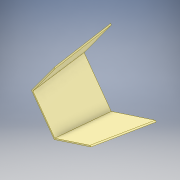
# Autodesk Inventor part: 花盆主体
Saved by Autodesk Inventor 2018 (Build 220112000, 112)
## iProperties
Created: 2021-02-25
Part Number: 花盆主体
Material: 尼龙 6/6
Document SubType Name: Modeling
Designer: OHHHHHHHHHH
Density: 1.13 g/cm^3
Appearance: 尼龙 6
Author: OHHHHHHHHHH
Autodesk Inventor part; units mm, degrees
sketch "草图1" plane through (0, 0, 0) normal (0, 1, 0) x (-1, 0, 0)
  line L0 (82.5131, 0) -> (25.498, -78.4746)
  line L1 (25.498, -78.4746) -> (-66.7545, -48.5)
  line L2 (-66.7545, -48.5) -> (-66.7545, 48.5)
  line L3 (-66.7545, 48.5) -> (25.498, 78.4746)
  line L4 (25.498, 78.4746) -> (82.5131, 0)
  point P0 (0, 0)
  point P1 (0, 0)
  dimension "d0" = 97
  constraints: 10 end point, 1 coincident, 11 other
  measures "d0" distance of L1.end L2.end
ref_plane "工作平面1" through (0, 170, 0) normal (0, 1, 0) x (-1, 0, 0)
sketch "草图2" plane through (0, 170, 0) normal (0, 1, 0) x (-1, 0, 0)
  line L0 (105.0554, 0) -> (32.4639, -99.9136)
  line L1 (32.4639, -99.9136) -> (-84.9916, -61.75)
  line L2 (-84.9916, -61.75) -> (-84.9916, 61.75)
  line L3 (-84.9916, 61.75) -> (32.4639, 99.9136)
  line L4 (32.4639, 99.9136) -> (105.0554, 0)
  point P0 (0, 0)
  point P1 (0, 0)
  dimension "d2" = 123.5
  constraints: 10 end point, 1 coincident, 11 other
  measures "d2" distance of L1.end L2.end
loft "放样1" add profiles "草图2", "草图1"
sketch "草图3" plane through (84.9916, 170, 61.75) normal (0, 1, 0) x (1, 0, 0)
  line L0 (-153.2988, 61.75) -> (-106.0997, 126.7141)
  line L1 (-106.0997, 126.7141) -> (-29.7298, 101.9)
  line L2 (-29.7298, 101.9) -> (-29.7298, 21.6)
  line L3 (-29.7298, 21.6) -> (-106.0997, -3.2141)
  line L4 (-106.0997, -3.2141) -> (-153.2988, 61.75)
  point P0 (-84.9916, 61.75)
  point P1 (-84.9916, 61.75)
  dimension "d7" = 80.3
  constraints: 10 end point, 1 coincident, 11 other
  measures "d7" distance of L1.end L2.end
extrude "拉伸1" cut sketch "草图3" against normal blind 164
shell "抽壳1" thickness 3 removed faces 1 at (10.4732, 170, -75.5426)
sketch "草图5" plane through (66.7545, 0, -48.5) normal (0, -1, 0) x (1, 0, 0)
  line L0 (-98.0659, 144.8667) -> (-91.2229, 123.806) projected
  line L1 (-106.5917, 71.5) -> (-123.9122, 81.5)
  line L2 (-107.7408, 69.3836) -> (-125.561, 78.4634)
  arc A0 (-106.5917, 71.5) -> (-107.7408, 69.3836) centre (-66.7545, 48.5) ccw
  arc A1 (-123.9122, 81.5) -> (-125.561, 78.4634) centre (-66.7545, 48.5) ccw
  point P0 (-99.2814, 81.0269)
  dimension "d37" = 132
  dimension "d38" = 92
  dimension "d40" = 3
  constraints: 5 point on circle, 4 end point, 2 centre point, 1 coincident
  measures "d37" diameter of A1
  measures "d38" diameter of A0
  measures "d40" angle of L1 L2
extrude "拉伸2" add sketch "草图5" along normal blind 3
sketch "草图7" plane through (66.7545, -3, -48.5) normal (0, -1, 0) x (1, 0, 0)
  arc A0 (-100.9392, 79.28) -> (-106.5917, 71.5) centre (-66.7545, 48.5) ccw
  arc A1 (-115.8021, 92.6626) -> (-125.561, 78.4634) centre (-66.7545, 48.5) ccw
  arc A2 (-100.9392, 79.28) -> (-107.7408, 69.3836) centre (-66.7545, 48.5) ccw
  line L0 (-100.9392, 79.28) -> (-115.8021, 92.6626)
  line L1 (-125.561, 78.4634) -> (-107.7408, 69.3836) projected
  line L2 (-107.7408, 69.3836) -> (-125.561, 78.4634)
  dimension "d25" = 92
  dimension "d41" = 15
  constraints: 6 point on circle, 4 end point, 3 centre point, 1 coincident, 1 collinear
  measures "d25" diameter of A0
  measures "d41" angle of L2 L0
extrude "拉伸3" add sketch "草图7" along normal blind 3
chamfer "倒角1" distance 1 angle 45 1 edges at (-41.6161, -3, 37.4713)
sketch "草图8" plane through (66.7545, 0, -48.5) normal (0, -1, 0) x (1, 0, 0)
  circle A0 centre (-66.7545, 48.5) radius 15
  dimension "d100" = 30
  constraints: 1 centre point, 1 coincident
  measures "d100" diameter of A0
extrude "拉伸4" add sketch "草图8" along normal blind 30
pattern_circular "环形阵列1" count 10 over 360 about axis through (0, -10, 0) along (0, 1, 0) of "拉伸3", "拉伸2", "倒角1"
sketch "草图9" plane through (64.0591, 3, 46.5417) normal (0, 1, 0) x (1, 0, 0)
  line L0 (-132.3664, 46.5417) -> (-85.1672, 111.5058) projected
  line L1 (-85.1672, -18.4224) -> (-132.3664, 46.5417) projected
  line L2 (-8.7974, 6.3917) -> (-85.1672, -18.4224) projected
  line L3 (-8.7974, 86.6917) -> (-8.7974, 6.3917) projected
  line L4 (-85.1672, 111.5058) -> (-8.7974, 86.6917) projected
  line L5 (-136.0746, 46.5417) -> (-86.3131, -21.9491) projected
  line L6 (-86.3131, -21.9491) -> (-5.7974, 4.2121) projected
  line L7 (-5.7974, 4.2121) -> (-5.7974, 88.8713) projected
  line L8 (-5.7974, 88.8713) -> (-86.3131, 115.0325) projected
  line L9 (-86.3131, 115.0325) -> (-136.0746, 46.5417) projected
  line L10 (-85.1672, -18.4224) -> (-132.3664, 46.5417) projected
  line L11 (-132.3664, 46.5417) -> (-85.1672, 111.5058) projected
  line L12 (-85.1672, 111.5058) -> (-8.7974, 86.6917) projected
  line L13 (-8.7974, 86.6917) -> (-8.7974, 6.3917) projected
  line L14 (-8.7974, 6.3917) -> (-85.1672, -18.4224) projected
  line L15 (-143.2406, 46.5417) -> (-88.5276, 121.8477) projected
  line L16 (-88.5276, -28.7643) -> (-143.2406, 46.5417) projected
  line L17 (0, 0) -> (-88.5276, -28.7643) projected
  line L18 (0, 93.0834) -> (0, 0) projected
  line L19 (-88.5276, 121.8477) -> (0, 93.0834) projected
  line L20 (-145.4076, 46.5417) -> (-89.1972, 123.9087)
  line L21 (-89.1972, 123.9087) -> (1.7532, 94.3571)
  line L22 (1.7532, 94.3571) -> (1.7532, -1.2738)
  line L23 (1.7532, -1.2738) -> (-89.1972, -30.8253)
  line L24 (-89.1972, -30.8253) -> (-145.4076, 46.5417)
  point P0 (-64.0591, 46.5417)
  constraints: 10 end point, 4 other
extrude "拉伸5" add sketch "草图9" along normal blind 15 contours L15 L19 L18 L17 L16 | L20 L21 L22 L23 L24
sketch "草图10" plane through (84.9916, 6, 61.75) normal (0, 1, 0) x (1, 0, 0)
  line L0 (-153.2988, 61.75) -> (-106.0997, 126.7141) projected
  line L1 (-106.0997, -3.2141) -> (-153.2988, 61.75) projected
  line L2 (-29.7298, 21.6) -> (-106.0997, -3.2141) projected
  line L3 (-29.7298, 101.9) -> (-29.7298, 21.6) projected
  line L4 (-106.0997, 126.7141) -> (-29.7298, 101.9) projected
  line L5 (-107.2456, 130.2408) -> (-157.007, 61.75) projected
  line L6 (-26.7298, 104.0796) -> (-107.2456, 130.2408) projected
  line L7 (-26.7298, 19.4204) -> (-26.7298, 104.0796) projected
  line L8 (-107.2456, -6.7408) -> (-26.7298, 19.4204) projected
  line L9 (-157.007, 61.75) -> (-107.2456, -6.7408) projected
  line L10 (-166.1621, 61.75) -> (-110.0746, 138.9477) projected
  line L11 (-110.0746, -15.4477) -> (-166.1621, 61.75) projected
  line L12 (-19.3233, 14.0392) -> (-110.0746, -15.4477) projected
  line L13 (-19.3233, 109.4608) -> (-19.3233, 14.0392) projected
  line L14 (-110.0746, 138.9477) -> (-19.3233, 109.4608) projected
  point P0 (-84.9916, 61.75)
sketch "草图11" plane through (64.0591, 18, 46.5417) normal (0, 1, 0) x (1, 0, 0)
  line L0 (-64.0591, 46.5417) -> (2.6954, 46.5417) construction
  line L1 (-86.3131, 115.0325) -> (-136.0746, 46.5417) projected
  line L2 (-5.7974, 88.8713) -> (-86.3131, 115.0325) projected
  line L3 (-5.7974, 4.2121) -> (-5.7974, 88.8713) projected
  line L4 (-86.3131, -21.9491) -> (-5.7974, 4.2121) projected
  line L5 (-136.0746, 46.5417) -> (-86.3131, -21.9491) projected
  line L6 (-145.2296, 46.5417) -> (-89.1422, 123.7394) projected
  line L7 (-89.1422, -30.656) -> (-145.2296, 46.5417) projected
  line L8 (1.6092, -1.1691) -> (-89.1422, -30.656) projected
  line L9 (1.6092, 94.2525) -> (1.6092, -1.1691) projected
  line L10 (-89.1422, 123.7394) -> (1.6092, 94.2525) projected
  circle A0 centre (-2.0908, 11.2121) radius 1.25
  line L11 (-5.7974, 4.2121) -> (1.6092, -1.1691) construction
  line L12 (-5.7974, 4.2121) -> (-5.7974, 88.8713) projected
  line L13 (-86.3131, -21.9491) -> (-5.7974, 4.2121) projected
  line L14 (1.6092, -1.1691) -> (-89.1422, -30.656) projected
  line L15 (1.6092, 94.2525) -> (1.6092, -1.1691) projected
  circle A1 centre (-11.3094, -1.4762) radius 1.25
  line L16 (-2.0941, 7.5215) -> (-0.5941, 7.5215)
  line L17 (-0.5941, 7.5215) -> (-0.5941, 0.4317)
  line L18 (-2.0941, 7.5215) -> (-3.5941, 7.5215)
  line L19 (-3.5941, 7.5215) -> (-3.5941, 2.6113)
  line L20 (-7.8005, -0.3326) -> (-7.3369, -1.7592)
  line L21 (-7.3369, -1.7592) -> (-0.5941, 0.4317)
  line L22 (-7.8005, -0.3326) -> (-8.264, 1.094)
  line L23 (-8.264, 1.094) -> (-3.5941, 2.6113)
  dimension "d63" = 2.5
  dimension "d69" = 3.7
  dimension "d131" = 3.6906
  constraints: 20 end point, 4 point on line, 4 symmetric about line, 2 centre point, 2 perpendicular, 1 other
  measures "d63" diameter of A0
  measures "d69" distance from line of L9 A0.centre
  measures "d131" distance from line of L22 A1.centre
extrude "拉伸7" cut sketch "草图11" against normal blind 3 contours A0 | A1 | L16 L17 L21 L20 L22 L23 L19 L18
extrude "拉伸8" add sketch "草图10" along normal blind 10 and the other way blind 3 contours L10 L14 L13 L12 L11
extrude "拉伸9" cut sketch "草图10" along normal blind 10 and the other way blind 3 contours L10 L14 L13 L12 L11
ref_plane "工作平面2" through (84.9916, 7, 61.75) normal (0, 1, 0) x (1, 0, 0)
sketch "草图12" plane through (84.9916, 7, 61.75) normal (0, 1, 0) x (1, 0, 0)
  line L0 (-107.2456, -6.7408) -> (-26.7298, 19.4204) projected
  line L1 (-60.7054, 8.3811) -> (-61.6324, 11.2342)
  line L2 (-29.7298, 21.6) -> (-106.0997, -3.2141) projected
  line L3 (-89.8404, 2.0689) -> (-88.9133, -0.7843)
  line L4 (-107.2456, -6.7408) -> (-26.7298, 19.4204) projected
  line L5 (-29.7298, 21.6) -> (-106.0997, -3.2141) projected
  line L6 (-63.5345, 10.6162) -> (-62.6075, 7.763)
  line L7 (-65.4366, 9.9982) -> (-64.5096, 7.145)
  line L8 (-67.3388, 9.3801) -> (-66.4117, 6.527)
  line L9 (-69.2409, 8.7621) -> (-68.3138, 5.9089)
  line L10 (-71.143, 8.1441) -> (-70.2159, 5.2909)
  line L11 (-73.0451, 7.526) -> (-72.118, 4.6729)
  line L12 (-74.9472, 6.908) -> (-74.0202, 4.0548)
  line L13 (-76.7905, 6.3091) -> (-75.7638, 3.4883)
  line L14 (-84.134, 3.923) -> (-83.207, 1.0698)
  line L15 (-86.0362, 3.305) -> (-85.1091, 0.4518)
  line L16 (-87.9383, 2.6869) -> (-87.0112, -0.1662)
  line L17 (-80.3298, 5.1591) -> (-79.4028, 2.3059)
  line L18 (-82.2319, 4.541) -> (-81.3049, 1.6879)
  line L19 (-78.4277, 5.7771) -> (-77.5006, 2.9239)
  line L20 (-61.6324, 11.2342) -> (-63.5345, 10.6162)
  line L21 (-62.6075, 7.763) -> (-60.7054, 8.3811)
  line L22 (-66.4117, 6.527) -> (-64.5096, 7.145)
  line L23 (-65.4366, 9.9982) -> (-67.3388, 9.3801)
  line L24 (-70.2159, 5.2909) -> (-68.3138, 5.9089)
  line L25 (-69.2409, 8.7621) -> (-71.143, 8.1441)
  line L26 (-74.0202, 4.0548) -> (-72.118, 4.6729)
  line L27 (-73.0451, 7.526) -> (-74.9472, 6.908)
  line L28 (-76.7905, 6.3091) -> (-78.4277, 5.7771)
  line L29 (-77.5006, 2.9239) -> (-75.7638, 3.4883)
  line L30 (-81.3049, 1.6879) -> (-79.4028, 2.3059)
  line L31 (-80.3298, 5.1591) -> (-82.2319, 4.541)
  line L32 (-84.134, 3.923) -> (-86.0362, 3.305)
  line L33 (-87.9383, 2.6869) -> (-89.8404, 2.0689)
  line L34 (-88.9133, -0.7843) -> (-87.0112, -0.1662)
  line L35 (-85.1091, 0.4518) -> (-83.207, 1.0698)
  line L36 (-58.8033, 8.9991) -> (-59.7303, 11.8523)
  line L37 (-56.9011, 9.6171) -> (-57.8282, 12.4703)
  line L38 (-54.999, 10.2352) -> (-55.9261, 13.0883)
  line L39 (-53.0969, 10.8532) -> (-54.024, 13.7064)
  point P0 (-84.9916, 61.75)
  dimension "d73" = 2
  dimension "d74" = 2
  dimension "d75" = 2
  dimension "d76" = 2
  dimension "d77" = 2
  dimension "d78" = 2
  dimension "d79" = 2
  dimension "d80" = 2
  dimension "d81" = 2
  dimension "d82" = 2
  dimension "d83" = 2
  dimension "d84" = 2
  dimension "d85" = 2
  dimension "d86" = 2
  dimension "d88" = 2
  dimension "d89" = 2
  dimension "d90" = 2
  dimension "d91" = 2
  constraints: 72 end point, 64 parallel, 50 perpendicular, 2 point on line, 40 other
  measures "d73" distance between parallel lines of L6 L1
  measures "d74" distance between parallel lines of L6 L7
  measures "d75" distance between parallel lines of L7 L8
  measures "d76" distance between parallel lines of L9 L8
  measures "d77" distance between parallel lines of L9 L10
  measures "d78" distance between parallel lines of L11 L12
  measures "d79" distance between parallel lines of L10 L11
  measures "d80" angle of L12 L13
  measures "d81" distance between parallel lines of L16 L3
  measures "d82" distance between parallel lines of L15 L16
  measures "d83" distance between parallel lines of L15 L14
  measures "d84" distance between parallel lines of L18 L14
  measures "d85" distance between parallel lines of L17 L18
  measures "d86" distance between parallel lines of L17 L19
  measures "d88" distance between parallel lines of L37 L38
  measures "d89" distance between parallel lines of L36 L1
  measures "d90" distance between parallel lines of L36 L37
  measures "d91" distance between parallel lines of L39 L38
extrude "拉伸10" cut sketch "草图12" along normal blind 7 contours L3 L2 L16 L0 | L15 L2 L14 L0 | L18 L2 L17 L0 | L19 L2 L13 L0 | L12 L2 L11 L0 | L10 L2 L9 L0 | L8 L2 L7 L0 | L6 L2 L1 L0 | L36 L2 L37 L0 | L38 L2 L39 L0
pattern_circular "环形阵列2" count 5 over 360 about axis through (0, 0, 0) along (0, -1, 0) of "拉伸10"
sketch "草图13" plane through (66.7545, 0, -48.5) normal (0, -1, 0) x (1, 0, 0)
  line L0 (1.9326, 98.4258) -> (-1.1068, 96.2175) construction
  line L1 (18.2371, 110.25) -> (0, 97) construction
  line L2 (-16.2555, 104.3138) -> (1.9326, 98.4258)
  line L3 (1.9326, 98.4258) -> (1.9326, 79.28)
  line L4 (-14.6399, 100.6147) -> (-1.1068, 96.2175)
  line L5 (-1.0862, 96.2108) -> (-1.0862, 81.9597)
  line L6 (-1.0862, 81.9597) -> (1.9326, 79.28)
  line L7 (-14.6399, 100.6147) -> (-16.2555, 104.3138)
  line L8 (1.9326, 98.4258) -> (1.9326, 79.28)
  line L9 (1.9326, 79.28) -> (-1.0862, 81.9597)
  line L10 (-1.0862, 0.7892) -> (-1.0862, 96.2108) projected
  line L11 (-1.0862, 81.9597) -> (-1.0862, 96.2108)
  line L12 (-1.0862, 96.2108) -> (-14.6399, 100.6147)
  line L13 (-91.8376, 125.6977) -> (-1.0862, 96.2108) projected
  line L14 (0, 97) -> (-92.2525, 126.9746) projected
  line L15 (-14.6399, 100.6147) -> (-16.2555, 104.3138)
  line L16 (-16.2555, 104.3138) -> (1.9326, 98.4258)
  point P0 (-66.7545, 48.5)
  point P1 (18.2371, 110.25)
  constraints: 26 end point, 5 collinear, 6 other
extrude "拉伸11" cut sketch "草图13" against normal blind 16
sketch "草图14" plane through (0, -30, 0) normal (0, -1, 0) x (1, 0, 0)
  line L0 (11.4602, -0.9019) -> (-11.5398, -0.9019)
  line L1 (-11.5398, -0.9019) -> (-11.5398, 0.7981)
  line L2 (-11.5398, 0.7981) -> (11.4602, 0.7981)
  line L3 (11.4602, 0.7981) -> (11.4602, -0.9019)
  line L4 (15.9292, -0.0519) -> (-16.622, -0.0519) construction
  line L5 (-0.0398, 4.6584) -> (-0.0398, -5.7431) construction
  point P0 (0, 0)
  dimension "d94" = 23
  dimension "d95" = 1.7
  constraints: 12 end point, 2 parallel, 1 horizontal, 1 perpendicular, 1 vertical, 2 other
  measures "d94" distance of L0.start L0.end
  measures "d95" distance of L0.end L1.end
extrude "拉伸12" cut sketch "草图14" along normal blind 10 and the other way blind 54.75
sketch "草图15" plane through (0, -30, 0) normal (0, -1, 0) x (1, 0, 0)
  line L0 (11.4602, 0.7981) -> (-11.5398, 0.7981) projected
  line L1 (9.9602, 0.7981) -> (-10.0398, 0.7981)
  line L2 (-10.0398, 0.7981) -> (-10.0398, 2.5981)
  line L3 (-10.0398, 2.5981) -> (9.9602, 2.5981)
  line L4 (9.9602, 2.5981) -> (9.9602, 0.7981)
  line L5 (11.4602, -0.9019) -> (-11.5398, -0.9019) projected
  line L6 (-0.0398, 30.3943) -> (-0.0398, -31.216) construction
  point P0 (0, 0)
  dimension "d101" = 3.5
  dimension "d102" = 20
  constraints: 10 end point, 2 parallel, 1 horizontal, 1 perpendicular, 1 point on line, 1 vertical, 1 other
  measures "d101" distance between parallel lines of L3 L5
  measures "d102" distance between parallel lines of L4 L2
extrude "拉伸13" cut sketch "草图15" against normal blind 30
sketch "草图16" plane through (0, -30, 0) normal (0, -1, 0) x (1, 0, 0)
  line L0 (11.4602, 0.7981) -> (-11.5398, 0.7981) projected
  line L1 (-5.5398, 0.7981) -> (5.4602, 0.7981)
  line L2 (5.4602, 0.7981) -> (5.4602, 6.5981)
  line L3 (5.4602, 6.5981) -> (-5.5398, 6.5981)
  line L4 (-5.5398, 6.5981) -> (-5.5398, 0.7981)
  line L5 (11.4602, -0.9019) -> (-11.5398, -0.9019) projected
  line L6 (-0.0398, 25.7819) -> (-0.0398, -22.2478) construction
  point P0 (0, 0)
  dimension "d105" = 7.5
  dimension "d106" = 11
  constraints: 10 end point, 2 parallel, 1 horizontal, 1 perpendicular, 1 point on line, 1 vertical, 1 other
  measures "d105" distance between parallel lines of L5 L3
  measures "d106" distance between parallel lines of L4 L2
extrude "拉伸14" cut sketch "草图16" against normal blind 6
ref_plane "工作平面3" through (0, -28, 0) normal (0, -1, 0) x (1, 0, 0)
sketch "草图18" plane through (0, -28, 0) normal (0, -1, 0) x (1, 0, 0)
  line L0 (5.4602, 6.5981) -> (5.4602, 2.5981) projected
  line L1 (5.4602, 2.5981) -> (9.9602, 2.5981) projected
  line L2 (9.9602, 2.5981) -> (9.9602, 0.7981) projected
  line L3 (9.9602, 0.7981) -> (11.4602, 0.7981) projected
  line L4 (11.4602, 0.7981) -> (11.4602, -0.9019) projected
  line L5 (11.4602, -0.9019) -> (-11.5398, -0.9019) projected
  line L6 (-11.5398, -0.9019) -> (-11.5398, 0.7981) projected
  line L7 (-11.5398, 0.7981) -> (-10.0398, 0.7981) projected
  line L8 (-10.0398, 0.7981) -> (-10.0398, 2.5981) projected
  line L9 (-10.0398, 2.5981) -> (-5.5398, 2.5981) projected
  line L10 (-5.5398, 2.5981) -> (-5.5398, 6.5981) projected
  line L11 (-5.5398, 6.5981) -> (5.4602, 6.5981) projected
  circle A0 centre (0, 0) radius 15 projected
  line L12 (-12.5398, -1.9019) -> (12.4602, -1.9019)
  line L13 (12.4602, -1.9019) -> (12.4602, 1.7981)
  line L14 (12.4602, 1.7981) -> (10.9602, 1.7981)
  line L15 (10.9602, 1.7981) -> (10.9602, 3.5981)
  line L16 (10.9602, 3.5981) -> (6.4602, 3.5981)
  line L17 (6.4602, 3.5981) -> (6.4602, 7.5981)
  line L18 (6.4602, 7.5981) -> (-6.5398, 7.5981)
  line L19 (-6.5398, 7.5981) -> (-6.5398, 3.5981)
  line L20 (-6.5398, 3.5981) -> (-11.0398, 3.5981)
  line L21 (-11.0398, 3.5981) -> (-11.0398, 1.7981)
  line L22 (-11.0398, 1.7981) -> (-12.5398, 1.7981)
  line L23 (-12.5398, 1.7981) -> (-12.5398, -1.9019)
  circle A1 centre (0, 0) radius 14
  point P0 (0, 0)
  dimension "d110" = 1
  dimension "d111" = 1
  constraints: 24 end point, 1 centre point, 11 other
  measures "d110" radial gap between concentric circles of A1 A0
  measures "d111" distance between parallel lines of L6 L23
extrude "拉伸15" cut sketch "草图18" against normal blind 30 contours A1
sketch "草图19" plane through (66.7545, 0, -48.5) normal (0, -1, 0) x (1, 0, 0)
  line L0 (-60.2943, 56.0981) -> (-73.2943, 56.0981) projected
  line L1 (-73.2943, 52.0981) -> (-77.7943, 52.0981) projected
  line L2 (-60.2943, 56.0981) -> (-73.2943, 56.0981)
  line L3 (-73.2943, 56.0981) -> (-73.2943, 52.0981)
  line L4 (-73.2943, 52.0981) -> (-60.2943, 52.0981)
  line L5 (-60.2943, 52.0981) -> (-60.2943, 56.0981)
  point P0 (-66.7545, 48.5)
  constraints: 8 end point, 2 parallel, 1 horizontal, 1 perpendicular
extrude "拉伸16" cut sketch "草图19" along normal blind 22 and the other way blind 2
sketch "草图21" plane through (0, -30, 0) normal (0, -1, 0) x (1, 0, 0)
  line L0 (5.4602, 6.5981) -> (5.4602, 2.5981) projected
  line L1 (5.4602, 2.5981) -> (9.9602, 2.5981) projected
  line L2 (9.9602, 2.5981) -> (9.9602, 0.7981) projected
  line L3 (9.9602, 0.7981) -> (11.4602, 0.7981) projected
  line L4 (11.4602, 0.7981) -> (11.4602, -0.9019) projected
  line L5 (11.4602, -0.9019) -> (-11.5398, -0.9019) projected
  line L6 (-11.5398, -0.9019) -> (-11.5398, 0.7981) projected
  line L7 (-11.5398, 0.7981) -> (-10.0398, 0.7981) projected
  line L8 (-10.0398, 0.7981) -> (-10.0398, 2.5981) projected
  line L9 (-10.0398, 2.5981) -> (-5.5398, 2.5981) projected
  line L10 (-5.5398, 2.5981) -> (-5.5398, 6.5981) projected
  line L11 (-5.5398, 6.5981) -> (5.4602, 6.5981) projected
  circle A0 centre (0, 0) radius 15 projected
  point P0 (0, 0)
extrude "拉伸17" add sketch "草图21" along normal blind 3
sketch "草图22" plane through (5.4602, -24, 6.5981) normal (0, 0, -1) x (-1, 0, 0)
  line L0 (9.1141, -4) -> (1.9525, -4)
  line L1 (1.9525, -4) -> (9.1141, -4)
  line L2 (9.1141, -4) -> (9.1141, -9.2971)
  line L3 (9.1141, -9.2971) -> (1.9525, -9.2971)
  line L4 (1.9525, -9.2971) -> (1.9525, -4)
  point P0 (5.4602, 24)
  constraints: 10 end point, 2 parallel, 1 horizontal, 1 perpendicular
extrude "拉伸18" cut sketch "草图22" against normal blind 10
sketch "草图23" plane through (0, -33, 0) normal (0, -1, 0) x (1, 0, 0)
  line L0 (5.555, -0.8779) -> (-5.9531, -0.8779)
  line L1 (-5.9531, -0.8779) -> (-5.9531, -3.3779)
  line L2 (-5.9531, -3.3779) -> (5.555, -3.3779)
  line L3 (5.555, -3.3779) -> (5.555, -0.8779)
  point P0 (0, 0)
  dimension "d125" = 2.5
  constraints: 8 end point, 2 parallel, 1 horizontal, 1 perpendicular
  measures "d125" distance between parallel lines of L2 L0
extrude "拉伸19" cut sketch "草图23" against normal blind 10
sketch "草图24" plane through (64.0591, 18, 46.5417) normal (0, 1, 0) x (1, 0, 0)
  line L0 (-75.5989, 45.7436) -> (-75.5989, 47.4436) projected
  line L1 (-75.5989, 47.4436) -> (-52.5989, 47.4436) projected
  line L2 (-52.5989, 47.4436) -> (-52.5989, 45.7436) projected
  line L3 (-52.5989, 45.7436) -> (-75.5989, 45.7436) projected
  line L4 (-132.3664, 46.5417) -> (-85.1672, 111.5058) projected
  line L5 (-85.1672, -18.4224) -> (-132.3664, 46.5417) projected
  line L6 (-8.7974, 6.3917) -> (-85.1672, -18.4224) projected
  line L7 (-8.7974, 86.6917) -> (-8.7974, 6.3917) projected
  line L8 (-85.1672, 111.5058) -> (-8.7974, 86.6917) projected
  line L9 (-2.9869, 2.1701) -> (-87.3867, -25.2531)
  line L10 (-87.3867, -25.2531) -> (-139.5486, 46.5417)
  line L11 (-139.5486, 46.5417) -> (-87.3867, 118.3364)
  line L12 (-87.3867, 118.3364) -> (-2.9869, 90.9133)
  line L13 (-2.9869, 90.9133) -> (-2.9869, 2.1701)
  line L14 (36.2149, -26.3117) -> (-102.3604, -71.3375)
  line L15 (-102.3604, -71.3375) -> (-188.0047, 46.5417)
  line L16 (-188.0047, 46.5417) -> (-102.3604, 164.4209)
  line L17 (-102.3604, 164.4209) -> (36.2149, 119.3951)
  line L18 (36.2149, 119.3951) -> (36.2149, -26.3117)
  point P0 (-64.0591, 46.5417)
  constraints: 20 end point, 8 other
extrude "拉伸20" cut sketch "草图24" along normal blind 1000 contours L14 L15 L16 L17 L18 keep common part
sketch "草图25" plane through (84.9916, 170, 61.75) normal (0, 1, 0) x (1, 0, 0)
  line L0 (0, 0) -> (-117.4555, -38.1636) projected
  line L1 (-84.9916, 61.75) -> (-117.4555, -38.1636)
  line L2 (-117.4555, -38.1636) -> (-259.2708, 40.5435)
  line L3 (-259.2708, 40.5435) -> (-138.2007, 195.9296)
  line L4 (-138.2007, 195.9296) -> (51.1158, 164.3125)
  line L5 (-117.4555, 161.6636) -> (0, 123.5) projected
  line L6 (51.1158, 164.3125) -> (0, 123.5)
  line L7 (0, 123.5) -> (-84.9916, 61.75)
  constraints: 12 end point
extrude "拉伸21" cut sketch "草图25" against normal blind 300 keep common part
